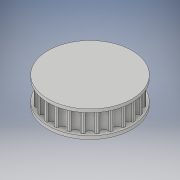
# Autodesk Inventor part: ParametricPulley
Saved by Autodesk Inventor 2019 (Build 230136000, 136)
## iProperties
Created: 2020-03-14
Part Number: ParametricPulley
Material: Generic
Document SubType Name: Modeling
Designer: gfellows
Density: 1 g/cm^3
Appearance: Default
Author: gfellows
Autodesk Inventor part; units mm, degrees
ref_plane "YZ Plane" through (0, 0, 0) normal (1, 0, 0) x (0, 1, 0)
ref_plane "XZ Plane" through (0, 0, 0) normal (0, 1, 0) x (-1, 0, 0)
ref_plane "XY Plane" through (0, 0, 0) normal (0, 0, 1) x (1, 0, 0)
sketch "Sketch1" plane through (0, 0, 0) normal (0, 1, 0) x (-1, 0, 0)
  circle A0 centre (0, 0) radius 18.5277 construction
  circle A1 centre (0, 0) radius 16.4677 construction
  line L0 (0, 0) -> (18.5277, 0) construction
  circle A2 centre (17.9927, 0) radius 1.525 construction
  circle A3 centre (17.9918, -1.955) radius 0.43 construction
  line L1 (0, 0) -> (17.8963, -4.7953) construction
  circle A4 centre (17.3796, -4.6568) radius 1.525 construction
  circle A5 centre (17.8847, -2.7682) radius 0.43 construction
  line L2 (0, 0) -> (16.4677, 0)
  line L3 (0, 0) -> (15.9065, -4.2621)
  line L4 (18.3096, -2.834) -> (18.4192, -2.0015)
  arc A6 (17.7736, -3.1836) -> (15.9065, -4.2621) centre (17.3796, -4.6568) ccw
  arc A7 (17.7736, -3.1836) -> (18.3096, -2.834) centre (17.8847, -2.7682) ccw
  arc A8 (18.4192, -2.0015) -> (17.992, -1.525) centre (17.9918, -1.955) ccw
  arc A9 (16.4677, 0) -> (17.992, -1.525) centre (17.9927, 0) ccw
  line L5 (0, 0) -> (16.4677, 0)
  line L6 (0, 0) -> (15.9065, -4.2621)
  arc A10 (17.7736, -3.1836) -> (15.9065, -4.2621) centre (17.3796, -4.6568) ccw
  arc A11 (16.4677, 0) -> (17.992, -1.525) centre (17.9927, 0) ccw
  arc A12 (18.4192, -2.0015) -> (17.992, -1.525) centre (17.9918, -1.955) ccw
  arc A13 (17.7736, -3.1836) -> (18.3096, -2.834) centre (17.8847, -2.7682) ccw
  dimension "d0" = 37.0553
  dimension "d1" = 32.9353
  dimension "d2" = 3.05
  dimension "d3" = 0.86
  dimension "d4" = 15
  dimension "d5" = 3.05
  dimension "d6" = 0.86
  constraints: 30 point on circle, 14 centre point, 14 end point, 10 coincident, 4 point on line, 4 tangent, 2 collinear, 1 horizontal
  measures "d0" diameter of A0
  measures "d1" diameter of A1
  measures "d2" diameter of A2
  measures "d3" diameter of A3
  measures "d4" angle of L0 L1
  measures "d5" diameter of A4
  measures "d6" diameter of A5
extrude "Extrusion1" add sketch "Sketch1" along normal blind 9.3
pattern_circular "Circular Pattern1" count 24 over 360 about axis through (0, 0, 0) along (0, 1, 0) of "Extrusion1"
sketch "Sketch2" plane through (0, 9.3, 0) normal (0, 1, 0) x (1, 0, 0)
  circle A0 centre (0, 0) radius 19.5277
  dimension "d12" = 39.0553
  constraints: 1 centre point, 1 coincident
  measures "d12" diameter of A0
sketch "Sketch3" plane through (0, 0, 0) normal (0, -1, 0) x (1, 0, 0)
  circle A0 centre (0, 0) radius 19.5277
  dimension "d13" = 39.0553
  constraints: 1 centre point, 1 coincident
  measures "d13" diameter of A0
extrude "Extrusion2" add sketch "Sketch2" along normal blind 1.5
extrude "Extrusion4" add sketch "Sketch3" along normal blind 1.5
equation "\"d0\" = OutsideDiameter"
equation "\"d7\" = Height"
equation "\"ToothPitch\" = 5"
equation "\"PitchLineOffset\" = 0.5715"
equation "\"Pi\" = 3.1415"
equation "\"Height\" = 9.3"
equation "\"OutsideDiameter\" = 37.055313"
body "Solid1"
